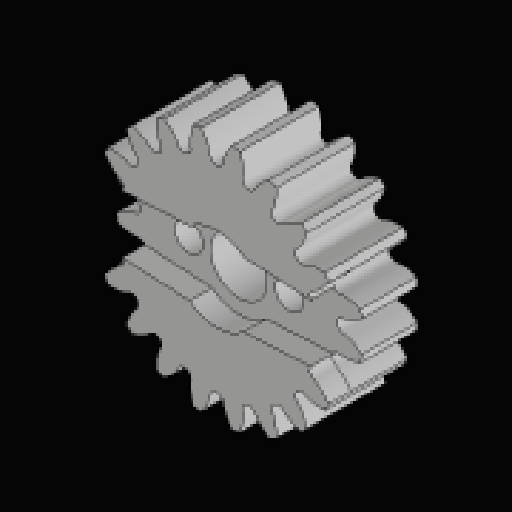
# Autodesk Inventor part: Servo Gear
Saved by Autodesk Inventor 2023.2 (Build 272271030, 271C)
## iProperties
Created: 2023-11-19
Part Number: Servo Gear
Material: Generic
Document SubType Name: Modeling
Designer: robpl
Density: 1 g/cm^3
Appearance: Default
Author: robpl
## iProperties of the stored document Servo Gear_3DPrint.ipt
Created: 2023-11-27
Part Number: Servo Gear_3DPrint
Material: Generic
Document SubType Name: Modeling
Designer: robpl
Density: 1 g/cm^3
Appearance: Default
Author: robpl
Autodesk Inventor part; units mm, degrees
ref_plane "YZ Plane" through (0, 0, 0) normal (1, 0, 0) x (0, 1, 0)
ref_plane "XZ Plane" through (0, 0, 0) normal (0, 1, 0) x (-1, 0, 0)
ref_plane "XY Plane" through (0, 0, 0) normal (0, 0, 1) x (1, 0, 0)
sketch "Sketch1" plane through (0, 0, 0) normal (0, 0, 1) x (1, 0, 0)
  spline S0 degree 3 poles (-1.3768, 10.9135) (-1.3419, 10.869) (-1.2721, 10.78) (-1.173, 10.6424) (-1.0781, 10.5017) (-0.9884, 10.3578) (-0.9041, 10.2106) (-0.826, 10.06) (-0.7548, 9.906) (-0.6919, 9.7484) (-0.6476, 9.6141) (-0.6191, 9.5046) (-0.6016, 9.4215) (-0.5932, 9.3371) (-0.5774, 9.2537) (-0.5568, 9.1714) (-0.5289, 9.0912) (-0.4924, 9.0144) (-0.4469, 8.9426) (-0.4, 8.8894) (-0.3582, 8.8513) (-0.3238, 8.8264) (-0.2881, 8.8034) (-0.2496, 8.7854) (-0.2102, 8.7696) (-0.169, 8.7594) (-0.1272, 8.7515) (-0.0706, 8.7491) (0, 8.7506) (0.0706, 8.7491) (0.1272, 8.7515) (0.169, 8.7594) (0.2102, 8.7696) (0.2496, 8.7854) (0.2881, 8.8034) (0.3238, 8.8264) (0.3582, 8.8513) (0.4, 8.8894) (0.4469, 8.9426) (0.4924, 9.0144) (0.5289, 9.0912) (0.5568, 9.1714) (0.5774, 9.2537) (0.5932, 9.3371) (0.6016, 9.4215) (0.6191, 9.5046) (0.6476, 9.6141) (0.6919, 9.7484) (0.7548, 9.906) (0.826, 10.06) (0.9041, 10.2106) (0.9884, 10.3578) (1.0781, 10.5017) (1.173, 10.6424) (1.2721, 10.78) (1.3419, 10.869) (1.3768, 10.9135) knots 0 0 0 0 0.01696 0.03392 0.050881 0.067841 0.084801 0.101761 0.11872 0.135679 0.152636 0.161116 0.169595 0.178075 0.186555 0.195032 0.203511 0.211989 0.220465 0.228938 0.233179 0.237417 0.241658 0.245897 0.250137 0.254376 0.258616 0.262855 0.271335 0.279816 0.284054 0.288295 0.292534 0.296774 0.301013 0.305254 0.309492 0.313732 0.322205 0.330682 0.33916 0.347638 0.356116 0.364596 0.373076 0.381555 0.390034 0.406992 0.423951 0.44091 0.45787 0.47483 0.49179 0.50875 0.52571 0.54267 0.54267 0.54267 0.54267
  circle A0 centre (0, 0) radius 8.75 construction
  circle A1 centre (0, 0) radius 9.3969 construction
  circle A2 centre (0, 0) radius 10 construction
  circle A3 centre (0, 0) radius 11
  point P0 (-1.2731, 10.7793)
  point P1 (-1.1737, 10.6419)
  point P2 (-1.079, 10.5012)
  point P3 (-0.9893, 10.3573)
  point P4 (-0.9051, 10.21)
  point P5 (-0.8271, 10.0594)
  point P6 (-0.7562, 9.9054)
  point P7 (-0.6935, 9.7478)
  point P8 (-0.641, 9.5865)
  point P9 (-0.6197, 9.5045)
  point P10 (-0.6031, 9.4213)
  point P11 (-0.592, 9.3373)
  point P12 (-0.5766, 9.2539)
  point P13 (-0.5556, 9.1717)
  point P14 (-0.5275, 9.0917)
  point P15 (-0.4909, 9.0153)
  point P16 (-0.4451, 8.9439)
  point P17 (-0.3892, 8.8802)
  point P18 (-0.3577, 8.8519)
  point P19 (-0.3236, 8.8267)
  point P20 (-0.2876, 8.8042)
  point P21 (-0.2495, 8.7858)
  point P22 (-0.2099, 8.7705)
  point P23 (-0.1689, 8.7598)
  point P24 (-0.1271, 8.7525)
  point P25 (-0.0848, 8.75)
  point P26 (0, 8.75)
  point P27 (0.0848, 8.75)
  point P28 (0.1271, 8.7525)
  point P29 (0.1689, 8.7598)
  point P30 (0.2099, 8.7705)
  point P31 (0.2495, 8.7858)
  point P32 (0.2876, 8.8042)
  point P33 (0.3236, 8.8267)
  point P34 (0.3577, 8.8519)
  point P35 (0.3892, 8.8802)
  point P36 (0.4451, 8.9439)
  point P37 (0.4909, 9.0153)
  point P38 (0.5275, 9.0917)
  point P39 (0.5556, 9.1717)
  point P40 (0.5766, 9.2539)
  point P41 (0.592, 9.3373)
  point P42 (0.6031, 9.4213)
  point P43 (0.6197, 9.5045)
  point P44 (0.641, 9.5865)
  point P45 (0.6935, 9.7478)
  point P46 (0.7562, 9.9054)
  point P47 (0.8271, 10.0594)
  point P48 (0.9051, 10.21)
  point P49 (0.9893, 10.3573)
  point P50 (1.079, 10.5012)
  point P51 (1.1737, 10.6419)
  point P52 (1.2731, 10.7793)
  constraints: 4 centre point, 2 point on circle, 115 other
extrude "Extrusion1" add sketch "Sketch1" against normal blind 5
extrude "Extrusion2" cut sketch "Sketch1" against normal through all contours A3 S0 picked at (-0.172, 10.4001)
pattern_circular "Circular Pattern1" count 20 over 360 about axis through (0, 0, 0) along (0, 0, -1) of "Extrusion2"
sketch "Sketch2" plane through (0, 0, -5) normal (0, 0, -1) x (-1, 0, 0)
  line L0 (-4.45, 0) -> (4.45, 0)
  point P0 (0, 0)
  point P1 (0, 0)
  dimension "d7" = 8.9
  constraints: 3 coincident, 2 end point, 1 horizontal, 1 midpoint
  measures "d7" distance of L0.start L0.end
hole "Hole1" at (4.45, 0, -5) at (-4.45, 0, -5) direction (0, 0, 1) diameter 2.5 end through all start extended yes counterbore diameter 6 counterbore depth 2
sketch "Sketch3" plane through (0, 0, -5) normal (0, 0, -1) x (-1, 0, 0)
  point P0 (0, 0)
  point P1 (0, 0)
  constraints: 1 coincident
hole "Hole2" at (0, 0, -5) direction (0, 0, 1) diameter 5 end through all start extended yes
sketch "Sketch4" plane through (0, 0, 0) normal (0, 0, 1) x (1, 0, 0)
  line L0 (-8.7471, 2.2927) -> (-2.2091, 2.65)
  arc A0 (2.2091, 2.65) -> (-2.2091, 2.65) centre (0, 0) ccw
  line L1 (2.2091, 2.65) -> (8.6578, 2.2976)
  line L2 (-2.2091, -2.65) -> (-8.7471, -2.2927)
  arc A1 (-2.2091, -2.65) -> (2.2091, -2.65) centre (0, 0) ccw
  line L3 (8.6578, -2.2976) -> (2.2091, -2.65)
  line L4 (50.7062, 0) -> (50.7062, 0)
  line L5 (-52.4366, -0.0945) -> (-52.4366, -0.0945)
  circle A2 centre (0, 0) radius 2.5
  circle A3 centre (4.45, 0) radius 1.25
  circle A4 centre (-4.45, 0) radius 1.25
  spline S0 degree 3 poles (-2.063, 10.8048) (-2.0825, 10.7517) (-2.1213, 10.6455) (-2.1731, 10.484) (-2.2199, 10.3209) (-2.2608, 10.1563) (-2.2954, 9.9902) (-2.3232, 9.8229) (-2.3432, 9.6544) (-2.3544, 9.4851) (-2.355, 9.3436) (-2.3483, 9.2308) (-2.3393, 9.1463) (-2.3211, 9.0634) (-2.3104, 8.9792) (-2.3045, 8.8946) (-2.3063, 8.8096) (-2.3173, 8.7254) (-2.3384, 8.643) (-2.3665, 8.5779) (-2.3946, 8.5288) (-2.4196, 8.4945) (-2.4464, 8.4616) (-2.4775, 8.4326) (-2.51, 8.4053) (-2.5461, 8.3829) (-2.5833, 8.3625) (-2.6364, 8.3427) (-2.7041, 8.3223) (-2.7708, 8.2991) (-2.8254, 8.2838) (-2.8675, 8.2785) (-2.9099, 8.2754) (-2.9522, 8.2783) (-2.9944, 8.2835) (-3.0354, 8.2944) (-3.0758, 8.3074) (-3.1274, 8.3307) (-3.1884, 8.3668) (-3.2539, 8.4211) (-3.3123, 8.4828) (-3.3637, 8.5504) (-3.4087, 8.6224) (-3.4495, 8.6968) (-3.4836, 8.7745) (-3.5259, 8.8481) (-3.5868, 8.9434) (-3.6704, 9.0575) (-3.779, 9.1879) (-3.8942, 9.3124) (-4.0151, 9.4315) (-4.1407, 9.5454) (-4.2706, 9.6546) (-4.4043, 9.759) (-4.5411, 9.8593) (-4.6349, 9.9224) (-4.6819, 9.9539) knots 0 0 0 0 0.031253 0.062506 0.09376 0.125013 0.156266 0.187518 0.21877 0.25002 0.281268 0.296894 0.312519 0.328145 0.343771 0.359393 0.375018 0.39064 0.406259 0.421873 0.429688 0.437497 0.445312 0.453124 0.460937 0.468748 0.476562 0.484373 0.5 0.515627 0.523438 0.531252 0.539063 0.546876 0.554688 0.562503 0.570312 0.578127 0.593741 0.60936 0.624982 0.640607 0.656229 0.671855 0.687481 0.703106 0.718732 0.74998 0.78123 0.812482 0.843734 0.874987 0.90624 0.937494 0.968747 1 1 1 1
  arc A5 (-4.6819, 9.9539) -> (-5.3009, 9.6385) centre (0, 0) ccw
  spline S1 degree 3 poles (-5.3009, 9.6385) (-5.303, 9.582) (-5.3072, 9.469) (-5.3064, 9.2993) (-5.3006, 9.1298) (-5.2886, 8.9606) (-5.2702, 8.7919) (-5.2449, 8.6242) (-5.2119, 8.4578) (-5.1702, 8.2933) (-5.1271, 8.1586) (-5.0858, 8.0533) (-5.0511, 7.9758) (-5.0083, 7.9025) (-4.9721, 7.8258) (-4.9403, 7.7471) (-4.9158, 7.6658) (-4.9002, 7.5823) (-4.8948, 7.4974) (-4.9014, 7.4268) (-4.9129, 7.3714) (-4.9261, 7.331) (-4.9414, 7.2914) (-4.962, 7.2543) (-4.9846, 7.2183) (-5.0119, 7.1858) (-5.041, 7.1549) (-5.0854, 7.1197) (-5.1435, 7.0794) (-5.1997, 7.0366) (-5.2469, 7.0053) (-5.2853, 6.9872) (-5.3247, 6.9712) (-5.3659, 6.9609) (-5.4076, 6.9528) (-5.45, 6.9504) (-5.4924, 6.9503) (-5.5487, 6.9565) (-5.6179, 6.972) (-5.6969, 7.0034) (-5.7715, 7.044) (-5.8413, 7.0925) (-5.9063, 7.147) (-5.9681, 7.2052) (-6.0246, 7.2686) (-6.0875, 7.3255) (-6.1749, 7.3973) (-6.2897, 7.48) (-6.4332, 7.5704) (-6.5813, 7.6532) (-6.733, 7.7291) (-6.8878, 7.7987) (-7.045, 7.8624) (-7.2044, 7.9204) (-7.3655, 7.9735) (-7.4743, 8.0045) (-7.5287, 8.0199) knots 0 0 0 0 0.031253 0.062506 0.09376 0.125013 0.156266 0.187518 0.21877 0.25002 0.281268 0.296894 0.312519 0.328145 0.343771 0.359393 0.375018 0.39064 0.406259 0.421873 0.429688 0.437497 0.445312 0.453124 0.460937 0.468748 0.476562 0.484373 0.5 0.515627 0.523438 0.531252 0.539063 0.546876 0.554688 0.562503 0.570312 0.578127 0.593741 0.60936 0.624982 0.640607 0.656229 0.671855 0.687481 0.703106 0.718732 0.74998 0.78123 0.812482 0.843734 0.874987 0.90624 0.937494 0.968747 1 1 1 1
  arc A6 (-7.5287, 8.0199) -> (-8.0199, 7.5287) centre (0, 0) ccw
  spline S2 degree 3 poles (-8.0199, 7.5287) (-8.0045, 7.4743) (-7.9735, 7.3655) (-7.9204, 7.2044) (-7.8624, 7.045) (-7.7987, 6.8878) (-7.7291, 6.733) (-7.6532, 6.5813) (-7.5704, 6.4332) (-7.48, 6.2897) (-7.3973, 6.1749) (-7.3255, 6.0875) (-7.2686, 6.0246) (-7.2052, 5.9681) (-7.147, 5.9063) (-7.0925, 5.8413) (-7.044, 5.7715) (-7.0034, 5.6969) (-6.972, 5.6179) (-6.9565, 5.5487) (-6.9503, 5.4924) (-6.9504, 5.45) (-6.9528, 5.4076) (-6.9609, 5.3659) (-6.9712, 5.3247) (-6.9872, 5.2853) (-7.0053, 5.2469) (-7.0366, 5.1997) (-7.0794, 5.1435) (-7.1197, 5.0854) (-7.1549, 5.041) (-7.1858, 5.0119) (-7.2183, 4.9846) (-7.2543, 4.962) (-7.2914, 4.9414) (-7.331, 4.9261) (-7.3714, 4.9129) (-7.4268, 4.9014) (-7.4974, 4.8948) (-7.5823, 4.9002) (-7.6658, 4.9158) (-7.7471, 4.9403) (-7.8258, 4.9721) (-7.9025, 5.0083) (-7.9758, 5.0511) (-8.0533, 5.0858) (-8.1586, 5.1271) (-8.2933, 5.1702) (-8.4578, 5.2119) (-8.6242, 5.2449) (-8.7919, 5.2702) (-8.9606, 5.2886) (-9.1298, 5.3006) (-9.2993, 5.3064) (-9.469, 5.3072) (-9.582, 5.303) (-9.6385, 5.3009) knots 0 0 0 0 0.031253 0.062506 0.09376 0.125013 0.156266 0.187518 0.21877 0.25002 0.281268 0.296894 0.312519 0.328145 0.343771 0.359393 0.375018 0.39064 0.406259 0.421873 0.429688 0.437497 0.445312 0.453124 0.460937 0.468748 0.476562 0.484373 0.5 0.515627 0.523438 0.531252 0.539063 0.546876 0.554688 0.562503 0.570312 0.578127 0.593741 0.60936 0.624982 0.640607 0.656229 0.671855 0.687481 0.703106 0.718732 0.74998 0.78123 0.812482 0.843734 0.874987 0.90624 0.937494 0.968747 1 1 1 1
  arc A7 (-9.6385, 5.3009) -> (-9.9539, 4.6819) centre (0, 0) ccw
  spline S3 degree 3 poles (-9.9539, 4.6819) (-9.9224, 4.6349) (-9.8593, 4.5411) (-9.759, 4.4043) (-9.6546, 4.2706) (-9.5454, 4.1407) (-9.4315, 4.0151) (-9.3124, 3.8942) (-9.1879, 3.779) (-9.0575, 3.6704) (-8.9434, 3.5868) (-8.8481, 3.5259) (-8.7745, 3.4836) (-8.6968, 3.4495) (-8.6224, 3.4087) (-8.5504, 3.3637) (-8.4828, 3.3123) (-8.4211, 3.2539) (-8.3668, 3.1884) (-8.3307, 3.1274) (-8.3074, 3.0758) (-8.2944, 3.0354) (-8.2835, 2.9944) (-8.2783, 2.9522) (-8.2754, 2.9099) (-8.2785, 2.8675) (-8.2838, 2.8254) (-8.2991, 2.7708) (-8.3223, 2.7041) (-8.3427, 2.6364) (-8.3625, 2.5833) (-8.3829, 2.5461) (-8.4053, 2.51) (-8.4326, 2.4775) (-8.4616, 2.4464) (-8.4945, 2.4196) (-8.5288, 2.3946) (-8.5779, 2.3665) (-8.643, 2.3384) (-8.7254, 2.3173) (-8.8096, 2.3063) (-8.8946, 2.3045) (-8.9792, 2.3104) (-9.0634, 2.3211) (-9.1463, 2.3393) (-9.2308, 2.3483) (-9.3436, 2.355) (-9.4851, 2.3544) (-9.6544, 2.3432) (-9.8229, 2.3232) (-9.9902, 2.2954) (-10.1563, 2.2608) (-10.3209, 2.2199) (-10.484, 2.1731) (-10.6455, 2.1213) (-10.7517, 2.0825) (-10.8048, 2.063) knots 0 0 0 0 0.031253 0.062506 0.09376 0.125013 0.156266 0.187518 0.21877 0.25002 0.281268 0.296894 0.312519 0.328145 0.343771 0.359393 0.375018 0.39064 0.406259 0.421873 0.429688 0.437497 0.445312 0.453124 0.460937 0.468748 0.476562 0.484373 0.5 0.515627 0.523438 0.531252 0.539063 0.546876 0.554688 0.562503 0.570312 0.578127 0.593741 0.60936 0.624982 0.640607 0.656229 0.671855 0.687481 0.703106 0.718732 0.74998 0.78123 0.812482 0.843734 0.874987 0.90624 0.937494 0.968747 1 1 1 1
  arc A8 (-10.8048, 2.063) -> (-10.9135, 1.3768) centre (0, 0) ccw
  arc A9 (-10.9135, -1.3768) -> (-10.8048, -2.063) centre (0, 0) ccw
  spline S4 degree 3 poles (-10.8048, -2.063) (-10.7517, -2.0825) (-10.6455, -2.1213) (-10.484, -2.1731) (-10.3209, -2.2199) (-10.1563, -2.2608) (-9.9902, -2.2954) (-9.8229, -2.3232) (-9.6544, -2.3432) (-9.4851, -2.3544) (-9.3436, -2.355) (-9.2308, -2.3483) (-9.1463, -2.3393) (-9.0634, -2.3211) (-8.9792, -2.3104) (-8.8946, -2.3045) (-8.8096, -2.3063) (-8.7254, -2.3173) (-8.643, -2.3384) (-8.5779, -2.3665) (-8.5288, -2.3946) (-8.4945, -2.4196) (-8.4616, -2.4464) (-8.4326, -2.4775) (-8.4053, -2.51) (-8.3829, -2.5461) (-8.3625, -2.5833) (-8.3427, -2.6364) (-8.3223, -2.7041) (-8.2991, -2.7708) (-8.2838, -2.8254) (-8.2785, -2.8675) (-8.2754, -2.9099) (-8.2783, -2.9522) (-8.2835, -2.9944) (-8.2944, -3.0354) (-8.3074, -3.0758) (-8.3307, -3.1274) (-8.3668, -3.1884) (-8.4211, -3.2539) (-8.4828, -3.3123) (-8.5504, -3.3637) (-8.6224, -3.4087) (-8.6968, -3.4495) (-8.7745, -3.4836) (-8.8481, -3.5259) (-8.9434, -3.5868) (-9.0575, -3.6704) (-9.1879, -3.779) (-9.3124, -3.8942) (-9.4315, -4.0151) (-9.5454, -4.1407) (-9.6546, -4.2706) (-9.759, -4.4043) (-9.8593, -4.5411) (-9.9224, -4.6349) (-9.9539, -4.6819) knots 0 0 0 0 0.031253 0.062506 0.09376 0.125013 0.156266 0.187518 0.21877 0.25002 0.281268 0.296894 0.312519 0.328145 0.343771 0.359393 0.375018 0.39064 0.406259 0.421873 0.429688 0.437497 0.445312 0.453124 0.460937 0.468748 0.476562 0.484373 0.5 0.515627 0.523438 0.531252 0.539063 0.546876 0.554688 0.562503 0.570312 0.578127 0.593741 0.60936 0.624982 0.640607 0.656229 0.671855 0.687481 0.703106 0.718732 0.74998 0.78123 0.812482 0.843734 0.874987 0.90624 0.937494 0.968747 1 1 1 1
  arc A10 (-9.9539, -4.6819) -> (-9.6385, -5.3009) centre (0, 0) ccw
  spline S5 degree 3 poles (-9.6385, -5.3009) (-9.582, -5.303) (-9.469, -5.3072) (-9.2993, -5.3064) (-9.1298, -5.3006) (-8.9606, -5.2886) (-8.7919, -5.2702) (-8.6242, -5.2449) (-8.4578, -5.2119) (-8.2933, -5.1702) (-8.1586, -5.1271) (-8.0533, -5.0858) (-7.9758, -5.0511) (-7.9025, -5.0083) (-7.8258, -4.9721) (-7.7471, -4.9403) (-7.6658, -4.9158) (-7.5823, -4.9002) (-7.4974, -4.8948) (-7.4268, -4.9014) (-7.3714, -4.9129) (-7.331, -4.9261) (-7.2914, -4.9414) (-7.2543, -4.962) (-7.2183, -4.9846) (-7.1858, -5.0119) (-7.1549, -5.041) (-7.1197, -5.0854) (-7.0794, -5.1435) (-7.0366, -5.1997) (-7.0053, -5.2469) (-6.9872, -5.2853) (-6.9712, -5.3247) (-6.9609, -5.3659) (-6.9528, -5.4076) (-6.9504, -5.45) (-6.9503, -5.4924) (-6.9565, -5.5487) (-6.972, -5.6179) (-7.0034, -5.6969) (-7.044, -5.7715) (-7.0925, -5.8413) (-7.147, -5.9063) (-7.2052, -5.9681) (-7.2686, -6.0246) (-7.3255, -6.0875) (-7.3973, -6.1749) (-7.48, -6.2897) (-7.5704, -6.4332) (-7.6532, -6.5813) (-7.7291, -6.733) (-7.7987, -6.8878) (-7.8624, -7.045) (-7.9204, -7.2044) (-7.9735, -7.3655) (-8.0045, -7.4743) (-8.0199, -7.5287) knots 0 0 0 0 0.031253 0.062506 0.09376 0.125013 0.156266 0.187518 0.21877 0.25002 0.281268 0.296894 0.312519 0.328145 0.343771 0.359393 0.375018 0.39064 0.406259 0.421873 0.429688 0.437497 0.445312 0.453124 0.460937 0.468748 0.476562 0.484373 0.5 0.515627 0.523438 0.531252 0.539063 0.546876 0.554688 0.562503 0.570312 0.578127 0.593741 0.60936 0.624982 0.640607 0.656229 0.671855 0.687481 0.703106 0.718732 0.74998 0.78123 0.812482 0.843734 0.874987 0.90624 0.937494 0.968747 1 1 1 1
  arc A11 (-8.0199, -7.5287) -> (-7.5287, -8.0199) centre (0, 0) ccw
  spline S6 degree 3 poles (-7.5287, -8.0199) (-7.4743, -8.0045) (-7.3655, -7.9735) (-7.2044, -7.9204) (-7.045, -7.8624) (-6.8878, -7.7987) (-6.733, -7.7291) (-6.5813, -7.6532) (-6.4332, -7.5704) (-6.2897, -7.48) (-6.1749, -7.3973) (-6.0875, -7.3255) (-6.0246, -7.2686) (-5.9681, -7.2052) (-5.9063, -7.147) (-5.8413, -7.0925) (-5.7715, -7.044) (-5.6969, -7.0034) (-5.6179, -6.972) (-5.5487, -6.9565) (-5.4924, -6.9503) (-5.45, -6.9504) (-5.4076, -6.9528) (-5.3659, -6.9609) (-5.3247, -6.9712) (-5.2853, -6.9872) (-5.2469, -7.0053) (-5.1997, -7.0366) (-5.1435, -7.0794) (-5.0854, -7.1197) (-5.041, -7.1549) (-5.0119, -7.1858) (-4.9846, -7.2183) (-4.962, -7.2543) (-4.9414, -7.2914) (-4.9261, -7.331) (-4.9129, -7.3714) (-4.9014, -7.4268) (-4.8948, -7.4974) (-4.9002, -7.5823) (-4.9158, -7.6658) (-4.9403, -7.7471) (-4.9721, -7.8258) (-5.0083, -7.9025) (-5.0511, -7.9758) (-5.0858, -8.0533) (-5.1271, -8.1586) (-5.1702, -8.2933) (-5.2119, -8.4578) (-5.2449, -8.6242) (-5.2702, -8.7919) (-5.2886, -8.9606) (-5.3006, -9.1298) (-5.3064, -9.2993) (-5.3072, -9.469) (-5.303, -9.582) (-5.3009, -9.6385) knots 0 0 0 0 0.031253 0.062506 0.09376 0.125013 0.156266 0.187518 0.21877 0.25002 0.281268 0.296894 0.312519 0.328145 0.343771 0.359393 0.375018 0.39064 0.406259 0.421873 0.429688 0.437497 0.445312 0.453124 0.460937 0.468748 0.476562 0.484373 0.5 0.515627 0.523438 0.531252 0.539063 0.546876 0.554688 0.562503 0.570312 0.578127 0.593741 0.60936 0.624982 0.640607 0.656229 0.671855 0.687481 0.703106 0.718732 0.74998 0.78123 0.812482 0.843734 0.874987 0.90624 0.937494 0.968747 1 1 1 1
  arc A12 (-5.3009, -9.6385) -> (-4.6819, -9.9539) centre (0, 0) ccw
  spline S7 degree 3 poles (-4.6819, -9.9539) (-4.6349, -9.9224) (-4.5411, -9.8593) (-4.4043, -9.759) (-4.2706, -9.6546) (-4.1407, -9.5454) (-4.0151, -9.4315) (-3.8942, -9.3124) (-3.779, -9.1879) (-3.6704, -9.0575) (-3.5868, -8.9434) (-3.5259, -8.8481) (-3.4836, -8.7745) (-3.4495, -8.6968) (-3.4087, -8.6224) (-3.3637, -8.5504) (-3.3123, -8.4828) (-3.2539, -8.4211) (-3.1884, -8.3668) (-3.1274, -8.3307) (-3.0758, -8.3074) (-3.0354, -8.2944) (-2.9944, -8.2835) (-2.9522, -8.2783) (-2.9099, -8.2754) (-2.8675, -8.2785) (-2.8254, -8.2838) (-2.7708, -8.2991) (-2.7041, -8.3223) (-2.6364, -8.3427) (-2.5833, -8.3625) (-2.5461, -8.3829) (-2.51, -8.4053) (-2.4775, -8.4326) (-2.4464, -8.4616) (-2.4196, -8.4945) (-2.3946, -8.5288) (-2.3665, -8.5779) (-2.3384, -8.643) (-2.3173, -8.7254) (-2.3063, -8.8096) (-2.3045, -8.8946) (-2.3104, -8.9792) (-2.3211, -9.0634) (-2.3393, -9.1463) (-2.3483, -9.2308) (-2.355, -9.3436) (-2.3544, -9.4851) (-2.3432, -9.6544) (-2.3232, -9.8229) (-2.2954, -9.9902) (-2.2608, -10.1563) (-2.2199, -10.3209) (-2.1731, -10.484) (-2.1213, -10.6455) (-2.0825, -10.7517) (-2.063, -10.8048) knots 0 0 0 0 0.031253 0.062506 0.09376 0.125013 0.156266 0.187518 0.21877 0.25002 0.281268 0.296894 0.312519 0.328145 0.343771 0.359393 0.375018 0.39064 0.406259 0.421873 0.429688 0.437497 0.445312 0.453124 0.460937 0.468748 0.476562 0.484373 0.5 0.515627 0.523438 0.531252 0.539063 0.546876 0.554688 0.562503 0.570312 0.578127 0.593741 0.60936 0.624982 0.640607 0.656229 0.671855 0.687481 0.703106 0.718732 0.74998 0.78123 0.812482 0.843734 0.874987 0.90624 0.937494 0.968747 1 1 1 1
  arc A13 (-2.063, -10.8048) -> (-1.3768, -10.9135) centre (0, 0) ccw
  spline S8 degree 3 poles (-1.3768, -10.9135) (-1.3419, -10.869) (-1.2721, -10.78) (-1.173, -10.6424) (-1.0781, -10.5017) (-0.9884, -10.3578) (-0.9041, -10.2106) (-0.826, -10.06) (-0.7548, -9.906) (-0.6919, -9.7484) (-0.6476, -9.6141) (-0.6191, -9.5046) (-0.6016, -9.4215) (-0.5932, -9.3371) (-0.5774, -9.2537) (-0.5568, -9.1714) (-0.5289, -9.0912) (-0.4924, -9.0144) (-0.4469, -8.9426) (-0.4, -8.8894) (-0.3582, -8.8513) (-0.3238, -8.8264) (-0.2881, -8.8034) (-0.2496, -8.7854) (-0.2102, -8.7696) (-0.169, -8.7594) (-0.1272, -8.7515) (-0.0706, -8.7491) (0, -8.7506) (0.0706, -8.7491) (0.1272, -8.7515) (0.169, -8.7594) (0.2102, -8.7696) (0.2496, -8.7854) (0.2881, -8.8034) (0.3238, -8.8264) (0.3582, -8.8513) (0.4, -8.8894) (0.4469, -8.9426) (0.4924, -9.0144) (0.5289, -9.0912) (0.5568, -9.1714) (0.5774, -9.2537) (0.5932, -9.3371) (0.6016, -9.4215) (0.6191, -9.5046) (0.6476, -9.6141) (0.6919, -9.7484) (0.7548, -9.906) (0.826, -10.06) (0.9041, -10.2106) (0.9884, -10.3578) (1.0781, -10.5017) (1.173, -10.6424) (1.2721, -10.78) (1.3419, -10.869) (1.3768, -10.9135) knots 0 0 0 0 0.031253 0.062506 0.09376 0.125013 0.156266 0.187518 0.21877 0.25002 0.281268 0.296894 0.312519 0.328145 0.343771 0.359393 0.375018 0.39064 0.406259 0.421873 0.429688 0.437497 0.445312 0.453124 0.460937 0.468748 0.476562 0.484373 0.5 0.515627 0.523438 0.531252 0.539063 0.546876 0.554688 0.562503 0.570312 0.578127 0.593741 0.60936 0.624982 0.640607 0.656229 0.671855 0.687481 0.703106 0.718732 0.74998 0.78123 0.812482 0.843734 0.874987 0.90624 0.937494 0.968747 1 1 1 1
  arc A14 (1.3768, -10.9135) -> (2.063, -10.8048) centre (0, 0) ccw
  spline S9 degree 3 poles (2.063, -10.8048) (2.0825, -10.7517) (2.1213, -10.6455) (2.1731, -10.484) (2.2199, -10.3209) (2.2608, -10.1563) (2.2954, -9.9902) (2.3232, -9.8229) (2.3432, -9.6544) (2.3544, -9.4851) (2.355, -9.3436) (2.3483, -9.2308) (2.3393, -9.1463) (2.3211, -9.0634) (2.3104, -8.9792) (2.3045, -8.8946) (2.3063, -8.8096) (2.3173, -8.7254) (2.3384, -8.643) (2.3665, -8.5779) (2.3946, -8.5288) (2.4196, -8.4945) (2.4464, -8.4616) (2.4775, -8.4326) (2.51, -8.4053) (2.5461, -8.3829) (2.5833, -8.3625) (2.6364, -8.3427) (2.7041, -8.3223) (2.7708, -8.2991) (2.8254, -8.2838) (2.8675, -8.2785) (2.9099, -8.2754) (2.9522, -8.2783) (2.9944, -8.2835) (3.0354, -8.2944) (3.0758, -8.3074) (3.1274, -8.3307) (3.1884, -8.3668) (3.2539, -8.4211) (3.3123, -8.4828) (3.3637, -8.5504) (3.4087, -8.6224) (3.4495, -8.6968) (3.4836, -8.7745) (3.5259, -8.8481) (3.5868, -8.9434) (3.6704, -9.0575) (3.779, -9.1879) (3.8942, -9.3124) (4.0151, -9.4315) (4.1407, -9.5454) (4.2706, -9.6546) (4.4043, -9.759) (4.5411, -9.8593) (4.6349, -9.9224) (4.6819, -9.9539) knots 0 0 0 0 0.031253 0.062506 0.09376 0.125013 0.156266 0.187518 0.21877 0.25002 0.281268 0.296894 0.312519 0.328145 0.343771 0.359393 0.375018 0.39064 0.406259 0.421873 0.429688 0.437497 0.445312 0.453124 0.460937 0.468748 0.476562 0.484373 0.5 0.515627 0.523438 0.531252 0.539063 0.546876 0.554688 0.562503 0.570312 0.578127 0.593741 0.60936 0.624982 0.640607 0.656229 0.671855 0.687481 0.703106 0.718732 0.74998 0.78123 0.812482 0.843734 0.874987 0.90624 0.937494 0.968747 1 1 1 1
  arc A15 (4.6819, -9.9539) -> (5.3009, -9.6385) centre (0, 0) ccw
  spline S10 degree 3 poles (5.3009, -9.6385) (5.303, -9.582) (5.3072, -9.469) (5.3064, -9.2993) (5.3006, -9.1298) (5.2886, -8.9606) (5.2702, -8.7919) (5.2449, -8.6242) (5.2119, -8.4578) (5.1702, -8.2933) (5.1271, -8.1586) (5.0858, -8.0533) (5.0511, -7.9758) (5.0083, -7.9025) (4.9721, -7.8258) (4.9403, -7.7471) (4.9158, -7.6658) (4.9002, -7.5823) (4.8948, -7.4974) (4.9014, -7.4268) (4.9129, -7.3714) (4.9261, -7.331) (4.9414, -7.2914) (4.962, -7.2543) (4.9846, -7.2183) (5.0119, -7.1858) (5.041, -7.1549) (5.0854, -7.1197) (5.1435, -7.0794) (5.1997, -7.0366) (5.2469, -7.0053) (5.2853, -6.9872) (5.3247, -6.9712) (5.3659, -6.9609) (5.4076, -6.9528) (5.45, -6.9504) (5.4924, -6.9503) (5.5487, -6.9565) (5.6179, -6.972) (5.6969, -7.0034) (5.7715, -7.044) (5.8413, -7.0925) (5.9063, -7.147) (5.9681, -7.2052) (6.0246, -7.2686) (6.0875, -7.3255) (6.1749, -7.3973) (6.2897, -7.48) (6.4332, -7.5704) (6.5813, -7.6532) (6.733, -7.7291) (6.8878, -7.7987) (7.045, -7.8624) (7.2044, -7.9204) (7.3655, -7.9735) (7.4743, -8.0045) (7.5287, -8.0199) knots 0 0 0 0 0.031253 0.062506 0.09376 0.125013 0.156266 0.187518 0.21877 0.25002 0.281268 0.296894 0.312519 0.328145 0.343771 0.359393 0.375018 0.39064 0.406259 0.421873 0.429688 0.437497 0.445312 0.453124 0.460937 0.468748 0.476562 0.484373 0.5 0.515627 0.523438 0.531252 0.539063 0.546876 0.554688 0.562503 0.570312 0.578127 0.593741 0.60936 0.624982 0.640607 0.656229 0.671855 0.687481 0.703106 0.718732 0.74998 0.78123 0.812482 0.843734 0.874987 0.90624 0.937494 0.968747 1 1 1 1
  arc A16 (7.5287, -8.0199) -> (8.0199, -7.5287) centre (0, 0) ccw
  spline S11 degree 3 poles (8.0199, -7.5287) (8.0045, -7.4743) (7.9735, -7.3655) (7.9204, -7.2044) (7.8624, -7.045) (7.7987, -6.8878) (7.7291, -6.733) (7.6532, -6.5813) (7.5704, -6.4332) (7.48, -6.2897) (7.3973, -6.1749) (7.3255, -6.0875) (7.2686, -6.0246) (7.2052, -5.9681) (7.147, -5.9063) (7.0925, -5.8413) (7.044, -5.7715) (7.0034, -5.6969) (6.972, -5.6179) (6.9565, -5.5487) (6.9503, -5.4924) (6.9504, -5.45) (6.9528, -5.4076) (6.9609, -5.3659) (6.9712, -5.3247) (6.9872, -5.2853) (7.0053, -5.2469) (7.0366, -5.1997) (7.0794, -5.1435) (7.1197, -5.0854) (7.1549, -5.041) (7.1858, -5.0119) (7.2183, -4.9846) (7.2543, -4.962) (7.2914, -4.9414) (7.331, -4.9261) (7.3714, -4.9129) (7.4268, -4.9014) (7.4974, -4.8948) (7.5823, -4.9002) (7.6658, -4.9158) (7.7471, -4.9403) (7.8258, -4.9721) (7.9025, -5.0083) (7.9758, -5.0511) (8.0533, -5.0858) (8.1586, -5.1271) (8.2933, -5.1702) (8.4578, -5.2119) (8.6242, -5.2449) (8.7919, -5.2702) (8.9606, -5.2886) (9.1298, -5.3006) (9.2993, -5.3064) (9.469, -5.3072) (9.582, -5.303) (9.6385, -5.3009) knots 0 0 0 0 0.031253 0.062506 0.09376 0.125013 0.156266 0.187518 0.21877 0.25002 0.281268 0.296894 0.312519 0.328145 0.343771 0.359393 0.375018 0.39064 0.406259 0.421873 0.429688 0.437497 0.445312 0.453124 0.460937 0.468748 0.476562 0.484373 0.5 0.515627 0.523438 0.531252 0.539063 0.546876 0.554688 0.562503 0.570312 0.578127 0.593741 0.60936 0.624982 0.640607 0.656229 0.671855 0.687481 0.703106 0.718732 0.74998 0.78123 0.812482 0.843734 0.874987 0.90624 0.937494 0.968747 1 1 1 1
  arc A17 (9.6385, -5.3009) -> (9.9539, -4.6819) centre (0, 0) ccw
  spline S12 degree 3 poles (9.9539, -4.6819) (9.9224, -4.6349) (9.8593, -4.5411) (9.759, -4.4043) (9.6546, -4.2706) (9.5454, -4.1407) (9.4315, -4.0151) (9.3124, -3.8942) (9.1879, -3.779) (9.0575, -3.6704) (8.9434, -3.5868) (8.8481, -3.5259) (8.7745, -3.4836) (8.6968, -3.4495) (8.6224, -3.4087) (8.5504, -3.3637) (8.4828, -3.3123) (8.4211, -3.2539) (8.3668, -3.1884) (8.3307, -3.1274) (8.3074, -3.0758) (8.2944, -3.0354) (8.2835, -2.9944) (8.2783, -2.9522) (8.2754, -2.9099) (8.2785, -2.8675) (8.2838, -2.8254) (8.2991, -2.7708) (8.3223, -2.7041) (8.3427, -2.6364) (8.3625, -2.5833) (8.3829, -2.5461) (8.4053, -2.51) (8.4326, -2.4775) (8.4616, -2.4464) (8.4945, -2.4196) (8.5288, -2.3946) (8.5779, -2.3665) (8.643, -2.3384) (8.7254, -2.3173) (8.8096, -2.3063) (8.8946, -2.3045) (8.9792, -2.3104) (9.0634, -2.3211) (9.1463, -2.3393) (9.2308, -2.3483) (9.3436, -2.355) (9.4851, -2.3544) (9.6544, -2.3432) (9.8229, -2.3232) (9.9902, -2.2954) (10.1563, -2.2608) (10.3209, -2.2199) (10.484, -2.1731) (10.6455, -2.1213) (10.7517, -2.0825) (10.8048, -2.063) knots 0 0 0 0 0.031253 0.062506 0.09376 0.125013 0.156266 0.187518 0.21877 0.25002 0.281268 0.296894 0.312519 0.328145 0.343771 0.359393 0.375018 0.39064 0.406259 0.421873 0.429688 0.437497 0.445312 0.453124 0.460937 0.468748 0.476562 0.484373 0.5 0.515627 0.523438 0.531252 0.539063 0.546876 0.554688 0.562503 0.570312 0.578127 0.593741 0.60936 0.624982 0.640607 0.656229 0.671855 0.687481 0.703106 0.718732 0.74998 0.78123 0.812482 0.843734 0.874987 0.90624 0.937494 0.968747 1 1 1 1
  arc A18 (10.8048, -2.063) -> (10.9135, -1.3768) centre (0, 0) ccw
  arc A19 (10.9135, 1.3768) -> (10.8048, 2.063) centre (0, 0) ccw
  spline S13 degree 3 poles (10.8048, 2.063) (10.7517, 2.0825) (10.6455, 2.1213) (10.484, 2.1731) (10.3209, 2.2199) (10.1563, 2.2608) (9.9902, 2.2954) (9.8229, 2.3232) (9.6544, 2.3432) (9.4851, 2.3544) (9.3436, 2.355) (9.2308, 2.3483) (9.1463, 2.3393) (9.0634, 2.3211) (8.9792, 2.3104) (8.8946, 2.3045) (8.8096, 2.3063) (8.7254, 2.3173) (8.643, 2.3384) (8.5779, 2.3665) (8.5288, 2.3946) (8.4945, 2.4196) (8.4616, 2.4464) (8.4326, 2.4775) (8.4053, 2.51) (8.3829, 2.5461) (8.3625, 2.5833) (8.3427, 2.6364) (8.3223, 2.7041) (8.2991, 2.7708) (8.2838, 2.8254) (8.2785, 2.8675) (8.2754, 2.9099) (8.2783, 2.9522) (8.2835, 2.9944) (8.2944, 3.0354) (8.3074, 3.0758) (8.3307, 3.1274) (8.3668, 3.1884) (8.4211, 3.2539) (8.4828, 3.3123) (8.5504, 3.3637) (8.6224, 3.4087) (8.6968, 3.4495) (8.7745, 3.4836) (8.8481, 3.5259) (8.9434, 3.5868) (9.0575, 3.6704) (9.1879, 3.779) (9.3124, 3.8942) (9.4315, 4.0151) (9.5454, 4.1407) (9.6546, 4.2706) (9.759, 4.4043) (9.8593, 4.5411) (9.9224, 4.6349) (9.9539, 4.6819) knots 0 0 0 0 0.031253 0.062506 0.09376 0.125013 0.156266 0.187518 0.21877 0.25002 0.281268 0.296894 0.312519 0.328145 0.343771 0.359393 0.375018 0.39064 0.406259 0.421873 0.429688 0.437497 0.445312 0.453124 0.460937 0.468748 0.476562 0.484373 0.5 0.515627 0.523438 0.531252 0.539063 0.546876 0.554688 0.562503 0.570312 0.578127 0.593741 0.60936 0.624982 0.640607 0.656229 0.671855 0.687481 0.703106 0.718732 0.74998 0.78123 0.812482 0.843734 0.874987 0.90624 0.937494 0.968747 1 1 1 1
  arc A20 (9.9539, 4.6819) -> (9.6385, 5.3009) centre (0, 0) ccw
  spline S14 degree 3 poles (9.6385, 5.3009) (9.582, 5.303) (9.469, 5.3072) (9.2993, 5.3064) (9.1298, 5.3006) (8.9606, 5.2886) (8.7919, 5.2702) (8.6242, 5.2449) (8.4578, 5.2119) (8.2933, 5.1702) (8.1586, 5.1271) (8.0533, 5.0858) (7.9758, 5.0511) (7.9025, 5.0083) (7.8258, 4.9721) (7.7471, 4.9403) (7.6658, 4.9158) (7.5823, 4.9002) (7.4974, 4.8948) (7.4268, 4.9014) (7.3714, 4.9129) (7.331, 4.9261) (7.2914, 4.9414) (7.2543, 4.962) (7.2183, 4.9846) (7.1858, 5.0119) (7.1549, 5.041) (7.1197, 5.0854) (7.0794, 5.1435) (7.0366, 5.1997) (7.0053, 5.2469) (6.9872, 5.2853) (6.9712, 5.3247) (6.9609, 5.3659) (6.9528, 5.4076) (6.9504, 5.45) (6.9503, 5.4924) (6.9565, 5.5487) (6.972, 5.6179) (7.0034, 5.6969) (7.044, 5.7715) (7.0925, 5.8413) (7.147, 5.9063) (7.2052, 5.9681) (7.2686, 6.0246) (7.3255, 6.0875) (7.3973, 6.1749) (7.48, 6.2897) (7.5704, 6.4332) (7.6532, 6.5813) (7.7291, 6.733) (7.7987, 6.8878) (7.8624, 7.045) (7.9204, 7.2044) (7.9735, 7.3655) (8.0045, 7.4743) (8.0199, 7.5287) knots 0 0 0 0 0.031253 0.062506 0.09376 0.125013 0.156266 0.187518 0.21877 0.25002 0.281268 0.296894 0.312519 0.328145 0.343771 0.359393 0.375018 0.39064 0.406259 0.421873 0.429688 0.437497 0.445312 0.453124 0.460937 0.468748 0.476562 0.484373 0.5 0.515627 0.523438 0.531252 0.539063 0.546876 0.554688 0.562503 0.570312 0.578127 0.593741 0.60936 0.624982 0.640607 0.656229 0.671855 0.687481 0.703106 0.718732 0.74998 0.78123 0.812482 0.843734 0.874987 0.90624 0.937494 0.968747 1 1 1 1
  arc A21 (8.0199, 7.5287) -> (7.5287, 8.0199) centre (0, 0) ccw
  spline S15 degree 3 poles (7.5287, 8.0199) (7.4743, 8.0045) (7.3655, 7.9735) (7.2044, 7.9204) (7.045, 7.8624) (6.8878, 7.7987) (6.733, 7.7291) (6.5813, 7.6532) (6.4332, 7.5704) (6.2897, 7.48) (6.1749, 7.3973) (6.0875, 7.3255) (6.0246, 7.2686) (5.9681, 7.2052) (5.9063, 7.147) (5.8413, 7.0925) (5.7715, 7.044) (5.6969, 7.0034) (5.6179, 6.972) (5.5487, 6.9565) (5.4924, 6.9503) (5.45, 6.9504) (5.4076, 6.9528) (5.3659, 6.9609) (5.3247, 6.9712) (5.2853, 6.9872) (5.2469, 7.0053) (5.1997, 7.0366) (5.1435, 7.0794) (5.0854, 7.1197) (5.041, 7.1549) (5.0119, 7.1858) (4.9846, 7.2183) (4.962, 7.2543) (4.9414, 7.2914) (4.9261, 7.331) (4.9129, 7.3714) (4.9014, 7.4268) (4.8948, 7.4974) (4.9002, 7.5823) (4.9158, 7.6658) (4.9403, 7.7471) (4.9721, 7.8258) (5.0083, 7.9025) (5.0511, 7.9758) (5.0858, 8.0533) (5.1271, 8.1586) (5.1702, 8.2933) (5.2119, 8.4578) (5.2449, 8.6242) (5.2702, 8.7919) (5.2886, 8.9606) (5.3006, 9.1298) (5.3064, 9.2993) (5.3072, 9.469) (5.303, 9.582) (5.3009, 9.6385) knots 0 0 0 0 0.031253 0.062506 0.09376 0.125013 0.156266 0.187518 0.21877 0.25002 0.281268 0.296894 0.312519 0.328145 0.343771 0.359393 0.375018 0.39064 0.406259 0.421873 0.429688 0.437497 0.445312 0.453124 0.460937 0.468748 0.476562 0.484373 0.5 0.515627 0.523438 0.531252 0.539063 0.546876 0.554688 0.562503 0.570312 0.578127 0.593741 0.60936 0.624982 0.640607 0.656229 0.671855 0.687481 0.703106 0.718732 0.74998 0.78123 0.812482 0.843734 0.874987 0.90624 0.937494 0.968747 1 1 1 1
  arc A22 (5.3009, 9.6385) -> (4.6819, 9.9539) centre (0, 0) ccw
  spline S16 degree 3 poles (4.6819, 9.9539) (4.6349, 9.9224) (4.5411, 9.8593) (4.4043, 9.759) (4.2706, 9.6546) (4.1407, 9.5454) (4.0151, 9.4315) (3.8942, 9.3124) (3.779, 9.1879) (3.6704, 9.0575) (3.5868, 8.9434) (3.5259, 8.8481) (3.4836, 8.7745) (3.4495, 8.6968) (3.4087, 8.6224) (3.3637, 8.5504) (3.3123, 8.4828) (3.2539, 8.4211) (3.1884, 8.3668) (3.1274, 8.3307) (3.0758, 8.3074) (3.0354, 8.2944) (2.9944, 8.2835) (2.9522, 8.2783) (2.9099, 8.2754) (2.8675, 8.2785) (2.8254, 8.2838) (2.7708, 8.2991) (2.7041, 8.3223) (2.6364, 8.3427) (2.5833, 8.3625) (2.5461, 8.3829) (2.51, 8.4053) (2.4775, 8.4326) (2.4464, 8.4616) (2.4196, 8.4945) (2.3946, 8.5288) (2.3665, 8.5779) (2.3384, 8.643) (2.3173, 8.7254) (2.3063, 8.8096) (2.3045, 8.8946) (2.3104, 8.9792) (2.3211, 9.0634) (2.3393, 9.1463) (2.3483, 9.2308) (2.355, 9.3436) (2.3544, 9.4851) (2.3432, 9.6544) (2.3232, 9.8229) (2.2954, 9.9902) (2.2608, 10.1563) (2.2199, 10.3209) (2.1731, 10.484) (2.1213, 10.6455) (2.0825, 10.7517) (2.063, 10.8048) knots 0 0 0 0 0.031253 0.062506 0.09376 0.125013 0.156266 0.187518 0.21877 0.25002 0.281268 0.296894 0.312519 0.328145 0.343771 0.359393 0.375018 0.39064 0.406259 0.421873 0.429688 0.437497 0.445312 0.453124 0.460937 0.468748 0.476562 0.484373 0.5 0.515627 0.523438 0.531252 0.539063 0.546876 0.554688 0.562503 0.570312 0.578127 0.593741 0.60936 0.624982 0.640607 0.656229 0.671855 0.687481 0.703106 0.718732 0.74998 0.78123 0.812482 0.843734 0.874987 0.90624 0.937494 0.968747 1 1 1 1
  arc A23 (2.063, 10.8048) -> (1.3768, 10.9135) centre (0, 0) ccw
  spline S17 degree 3 poles (1.3768, 10.9135) (1.3419, 10.869) (1.2721, 10.78) (1.173, 10.6424) (1.0781, 10.5017) (0.9884, 10.3578) (0.9041, 10.2106) (0.826, 10.06) (0.7548, 9.906) (0.6919, 9.7484) (0.6476, 9.6141) (0.6191, 9.5046) (0.6016, 9.4215) (0.5932, 9.3371) (0.5774, 9.2537) (0.5568, 9.1714) (0.5289, 9.0912) (0.4924, 9.0144) (0.4469, 8.9426) (0.4, 8.8894) (0.3582, 8.8513) (0.3238, 8.8264) (0.2881, 8.8034) (0.2496, 8.7854) (0.2102, 8.7696) (0.169, 8.7594) (0.1272, 8.7515) (0.0706, 8.7491) (0, 8.7506) (-0.0706, 8.7491) (-0.1272, 8.7515) (-0.169, 8.7594) (-0.2102, 8.7696) (-0.2496, 8.7854) (-0.2881, 8.8034) (-0.3238, 8.8264) (-0.3582, 8.8513) (-0.4, 8.8894) (-0.4469, 8.9426) (-0.4924, 9.0144) (-0.5289, 9.0912) (-0.5568, 9.1714) (-0.5774, 9.2537) (-0.5932, 9.3371) (-0.6016, 9.4215) (-0.6191, 9.5046) (-0.6476, 9.6141) (-0.6919, 9.7484) (-0.7548, 9.906) (-0.826, 10.06) (-0.9041, 10.2106) (-0.9884, 10.3578) (-1.0781, 10.5017) (-1.173, 10.6424) (-1.2721, 10.78) (-1.3419, 10.869) (-1.3768, 10.9135) knots 0 0 0 0 0.031253 0.062506 0.09376 0.125013 0.156266 0.187518 0.21877 0.25002 0.281268 0.296894 0.312519 0.328145 0.343771 0.359393 0.375018 0.39064 0.406259 0.421873 0.429688 0.437497 0.445312 0.453124 0.460937 0.468748 0.476562 0.484373 0.5 0.515627 0.523438 0.531252 0.539063 0.546876 0.554688 0.562503 0.570312 0.578127 0.593741 0.60936 0.624982 0.640607 0.656229 0.671855 0.687481 0.703106 0.718732 0.74998 0.78123 0.812482 0.843734 0.874987 0.90624 0.937494 0.968747 1 1 1 1
  arc A24 (-1.3768, 10.9135) -> (-2.063, 10.8048) centre (0, 0) ccw
  circle A25 centre (0, 0) radius 3.75
  line L6 (2.389, -2.8905) -> (13, -2.3107)
  line L7 (13, -2.3107) -> (13, 2.3107)
  line L8 (13, 2.3107) -> (2.389, 2.8905)
  line L9 (-2.389, 2.8905) -> (-13, 2.3107)
  line L10 (-13, 2.3107) -> (-13, -2.3107)
  line L11 (-13, -2.3107) -> (-2.389, -2.8905)
  point P0 (-8.3735, 2.5635)
  point P1 (8.3735, 2.5635)
  point P2 (8.3735, -2.5635)
  point P3 (-8.3735, -2.5635)
extrude "Extrusion3" add sketch "Sketch4" along normal blind 2 contours L9 S3 A7 S2 A6 S1 A5 S0 A24 S17 A23 S16 A22 S15 A21 S14 A20 S13 L8 A25 | A25 L6 S12 A17 S11 A16 S10 A15 S9 A14 S8 A13 S7 A12 S6 A11 S5 A10 S4 L11
sketch "Sketch6" plane through (0, 0, 0) normal (0, 1, 0) x (-1, 0, 0)
  line L0 (-2.5, 0) -> (2.5, 0) projected
  line L1 (-1.916, -5) -> (-1.916, -3) projected
  line L2 (1.916, -5) -> (-1.916, -5) projected
  line L3 (1.916, -3) -> (1.916, -5) projected
  line L4 (1.916, -3) -> (1.916, -3) projected
  line L5 (1.916, -5) -> (1.916, -3) projected
  line L6 (-1.916, -5) -> (1.916, -5) projected
  line L7 (-1.916, -3) -> (-1.916, -5) projected
  line L8 (-1.916, -3) -> (-1.916, -3) projected
  line L9 (0, -5) -> (-11, -5)
  line L10 (-11, -5) -> (-11, -4.5)
  line L11 (-11, -4.5) -> (-10.5, -5)
  line L12 (0, -6.4043) -> (0, 3.4007) projected
  point P0 (0, 0)
  dimension "d33" = 11
  dimension "d34" = 0.5
  dimension "d35" = 0.5
  constraints: 6 end point, 2 point on line, 1 midpoint, 1 vertical
  measures "d33" distance of L9.start L9.end
  measures "d34" distance of L9.end L10.end
  measures "d35" distance of L11.end L9.end
revolve "Revolution2" cut sketch "Sketch6" angle 360 about axis through (0, 0, -10) along (0, 0, 1)
equation "\"d0\" = FaceWidth"
equation "\"d35\" = d34"
equation "\"Module\" = 1"
equation "\"PressureAngle\" = 20deg"
equation "\"UnitProfileClearance\" = 0.25"
equation "\"UnitRoundRadius\" = 0.35"
equation "\"HeadDiameter\" = 22"
equation "\"RootDiameter\" = 17.5"
equation "\"BaseDiameter\" = 18.79385"
equation "\"FaceWidth\" = 5"
equation "\"HelixAngle\" = 0"
equation "\"UnitCorrection\" = 0"
equation "\"UnitAddendumModification\" = 0"
equation "\"CircularPitch\" = 3.141593"
equation "\"UnitBacklashShift\" = 0"
equation "\"TotalToolShift\" = 0"
equation "\"IsInternal\" = 0"
equation "\"d24\" = d23"
equation "\"d25\" = d23"
equation "\"d26\" = d25"
equation "\"d23\" = 0.25"
body "Solid1"
